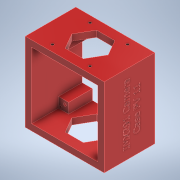
# Autodesk Inventor part: IMX291 Camera Case Base
Saved by Autodesk Inventor 2022.1 (Build 261234000, 234)
## iProperties
Created: 2021-07-23
Part Number: IMX291 Camera Case Base
Material: PET Plastic
Document SubType Name: Modeling
Designer: robst
Density: 1.541 g/cm^3
Appearance: Red
Author: robst
Autodesk Inventor part; units mm, degrees
ref_plane "YZ Plane" through (0, 0, 0) normal (1, 0, 0) x (0, 1, 0)
ref_plane "XZ Plane" through (0, 0, 0) normal (0, 1, 0) x (-1, 0, 0)
ref_plane "XY Plane" through (0, 0, 0) normal (0, 0, 1) x (1, 0, 0)
sketch "Sketch8" plane through (0, 0, 0) normal (0, 0, 1) x (1, 0, 0)
  line L0 (-17, -17) -> (17, -17) construction
  line L1 (17, -17) -> (17, 17) construction
  line L2 (17, 17) -> (-17, 17) construction
  line L3 (-17, 17) -> (-17, -17) construction
  line L4 (-17, -17) -> (17, 17) construction
  line L5 (17, -17) -> (-17, 17) construction
  circle A0 centre (-17, 17) radius 0.9
  circle A1 centre (17, 17) radius 0.9
  circle A2 centre (17, -17) radius 0.9
  circle A3 centre (-17, -17) radius 0.9
  line L6 (-21, -21) -> (21, -21)
  line L7 (21, -21) -> (21, 21)
  line L8 (21, 21) -> (-21, 21)
  line L9 (-21, 21) -> (-21, -21)
  line L10 (-21, -21) -> (21, 21) construction
  line L11 (21, -21) -> (-21, 21) construction
  line L12 (-25, -25) -> (25, -25)
  line L13 (25, -25) -> (25, 25)
  line L14 (25, 25) -> (-25, 25)
  line L15 (-25, 25) -> (-25, -25)
  line L16 (-25, -25) -> (25, 25) construction
  line L17 (25, -25) -> (-25, 25) construction
  line L18 (0, 0) -> (9.8286, 0)
  line L19 (-14.5, -14.5) -> (14.5, -14.5) construction
  line L20 (14.5, -14.5) -> (14.5, 14.5) construction
  line L21 (14.5, 14.5) -> (-14.5, 14.5) construction
  line L22 (-14.5, 14.5) -> (-14.5, -14.5) construction
  line L23 (-14.5, -14.5) -> (14.5, 14.5) construction
  line L24 (14.5, -14.5) -> (-14.5, 14.5) construction
  line L25 (-21, 21) -> (-14.5, 21)
  line L26 (-14.5, 21) -> (-14.5, 14.5)
  line L27 (-14.5, 14.5) -> (-21, 14.5)
  line L28 (-21, 14.5) -> (-21, 21)
  line L29 (21, 21) -> (14.5, 21)
  line L30 (14.5, 21) -> (14.5, 14.5)
  line L31 (14.5, 14.5) -> (21, 14.5)
  line L32 (21, 14.5) -> (21, 21)
  line L33 (21, -21) -> (14.5, -21)
  line L34 (14.5, -21) -> (14.5, -14.5)
  line L35 (14.5, -14.5) -> (21, -14.5)
  line L36 (21, -14.5) -> (21, -21)
  line L37 (-21, -21) -> (-14.5, -21)
  line L38 (-14.5, -21) -> (-14.5, -14.5)
  line L39 (-14.5, -14.5) -> (-21, -14.5)
  line L40 (-21, -14.5) -> (-21, -21)
  point P0 (-25, 0)
  point P1 (-14.5, -21)
  dimension "d46" = 34
  dimension "d47" = 34
  dimension "d48" = 1.8
  dimension "d49" = 42
  dimension "d50" = 42
  dimension "d51" = 4
  dimension "d52" = 4
  dimension "d53" = 29
  dimension "d54" = 29
  dimension "d61" = 50
  dimension "d62" = 50
  constraints: 82 end point, 16 parallel, 9 midpoint, 8 horizontal, 8 perpendicular, 4 centre point, 4 coincident, 3 equal radius, 2 point on line
  measures "d46" distance of L0.start L0.end
  measures "d47" distance of L2.end L0.start
  measures "d48" diameter of A0
  measures "d49" distance of L7.end L8.end
  measures "d50" distance of L6.end L7.end
  measures "d51" distance between parallel lines of L8 L14
  measures "d52" distance from line of point (-25, 0) L9
  measures "d53" distance of L19.start L19.end
  measures "d54" distance of L20.end L19.end
  measures "d61" distance between parallel lines of L14 L12
  measures "d62" distance between parallel lines of L15 L13
extrude "Extrusion9" add sketch "Sketch8" against normal blind 15 contours L9 L39 L38 L6 | L34 L35 L7 L6 | L9 L8 L26 L27 | L31 L30 L8 L7 | L15 L14 L13 L12
sketch "Sketch9" plane through (0, 0, 0) normal (0, 0, 1) x (1, 0, 0)
  line L0 (21, 14.5) -> (21, -14.5) projected
  line L1 (-14.5, 21) -> (14.5, 21) projected
  line L2 (-21, -14.5) -> (-21, 14.5) projected
  line L3 (14.5, -21) -> (-14.5, -21) projected
  line L4 (-25, -25) -> (25, -25) projected
  line L5 (25, -25) -> (25, 25) projected
  line L6 (25, 25) -> (-25, 25) projected
  line L7 (-25, 25) -> (-25, -25) projected
  line L8 (-21, -21) -> (21, -21)
  line L9 (21, -21) -> (21, 21)
  line L10 (21, 21) -> (-21, 21)
  line L11 (-21, 21) -> (-21, -21)
  line L12 (-21, -21) -> (21, 21) construction
  line L13 (21, -21) -> (-21, 21) construction
  line L14 (-23, -23) -> (23, -23)
  line L15 (23, -23) -> (23, 23)
  line L16 (23, 23) -> (-23, 23)
  line L17 (-23, 23) -> (-23, -23)
  line L18 (-23, -23) -> (23, 23) construction
  line L19 (23, -23) -> (-23, 23) construction
  point P0 (0, 0)
  point P1 (-14.5, -21)
  constraints: 24 end point, 4 midpoint, 4 parallel, 2 perpendicular
extrude "Extrusion10" add sketch "Sketch9" along normal blind 17 contours L7 L6 L5 L4 | L17 L16 L15 L14
sketch "Sketch10" plane through (25, -25, -15) normal (1, 0, 0) x (0, 0, -1)
  line L0 (-32, 0) -> (0, 0) construction
  line L1 (-16, 0) -> (-16, 50) construction
  line L2 (0, 50) -> (-32, 50) construction
  line L3 (-16, 7.4068) -> (-16, 5.8574)
  line L4 (-16, 5.8574) -> (-16.4084, 5.8574)
  line L5 (-16.4084, 5.8574) -> (-16.4084, 6.3663)
  line L6 (-16.4084, 6.3663) -> (-19.5916, 6.3663)
  line L7 (-19.5916, 6.3663) -> (-19.5916, 5.8574)
  line L8 (-19.5916, 5.8574) -> (-20, 5.8574)
  line L9 (-20, 5.8574) -> (-20, 7.4068)
  line L10 (-20, 7.4068) -> (-19.5916, 7.4068)
  line L11 (-19.5916, 7.4068) -> (-19.5916, 6.8979)
  line L12 (-19.5916, 6.8979) -> (-16.4084, 6.8979)
  line L13 (-16.4084, 6.8979) -> (-16.4084, 7.4068)
  line L14 (-16.4084, 7.4068) -> (-16, 7.4068)
  line L15 (-16, 11.4943) -> (-16, 10.9627)
  line L16 (-16, 10.9627) -> (-19.4457, 10.9627)
  line L17 (-19.4457, 10.9627) -> (-17.1021, 9.919)
  line L18 (-17.1021, 9.919) -> (-17.1021, 9.5948)
  line L19 (-17.1021, 9.5948) -> (-19.4457, 8.5608)
  line L20 (-19.4457, 8.5608) -> (-16, 8.5608)
  line L21 (-16, 8.5608) -> (-16, 8.0648)
  line L22 (-16, 8.0648) -> (-20, 8.0648)
  line L23 (-20, 8.0648) -> (-20, 8.7909)
  line L24 (-20, 8.7909) -> (-17.7731, 9.7893)
  line L25 (-17.7731, 9.7893) -> (-20, 10.7553)
  line L26 (-20, 10.7553) -> (-20, 11.4943)
  line L27 (-20, 11.4943) -> (-16, 11.4943)
  line L28 (-16, 15.0697) -> (-16, 14.4603)
  line L29 (-16, 14.4603) -> (-17.5948, 13.4878)
  line L30 (-17.5948, 13.4878) -> (-16, 12.4959)
  line L31 (-16, 12.4959) -> (-16, 11.9222)
  line L32 (-16, 11.9222) -> (-18.0032, 13.1961)
  line L33 (-18.0032, 13.1961) -> (-20, 11.9611)
  line L34 (-20, 11.9611) -> (-20, 12.5705)
  line L35 (-20, 12.5705) -> (-18.4344, 13.5235)
  line L36 (-18.4344, 13.5235) -> (-20, 14.4959)
  line L37 (-20, 14.4959) -> (-20, 15.0697)
  line L38 (-20, 15.0697) -> (-18.0292, 13.8185)
  line L39 (-18.0292, 13.8185) -> (-16, 15.0697)
  line L40 (-16, 17.8509) -> (-16, 15.3841)
  line L41 (-16, 15.3841) -> (-16.5673, 15.3841)
  spline S0 degree 2 poles (-16.5673, 15.3841) (-16.8169, 15.6499) (-17.2804, 16.1232) (-17.53, 16.3501) knots 0 0 0 1 2 2 2
  spline S1 degree 2 poles (-17.53, 16.3501) (-18.0324, 16.8071) (-18.6353, 17.141) (-18.9562, 17.141) knots 0 0 0 1 2 2 2
  spline S2 degree 2 poles (-18.9562, 17.141) (-19.1248, 17.141) (-19.3776, 17.0373) (-19.4587, 16.9433) knots 0 0 0 1 2 2 2
  spline S3 degree 2 poles (-19.4587, 16.9433) (-19.5397, 16.8493) (-19.6207, 16.6029) (-19.6207, 16.4538) knots 0 0 0 1 2 2 2
  spline S4 degree 2 poles (-19.6207, 16.4538) (-19.6207, 16.3112) (-19.5494, 16.0194) (-19.4943, 15.8865) knots 0 0 0 1 2 2 2
  spline S5 degree 2 poles (-19.4943, 15.8865) (-19.4489, 15.7731) (-19.3193, 15.5624) (-19.2739, 15.4976) knots 0 0 0 1 2 2 2
  line L42 (-19.2739, 15.4976) -> (-19.2739, 15.4684)
  line L43 (-19.2739, 15.4684) -> (-19.8444, 15.4684)
  spline S6 degree 2 poles (-19.8444, 15.4684) (-19.9254, 15.6337) (-20.0843, 16.2269) (-20.0843, 16.4927) knots 0 0 0 1 2 2 2
  spline S7 degree 2 poles (-20.0843, 16.4927) (-20.0843, 17.0535) (-19.4911, 17.6856) (-18.9854, 17.6856) knots 0 0 0 1 2 2 2
  spline S8 degree 2 poles (-18.9854, 17.6856) (-18.7488, 17.6856) (-18.3533, 17.5754) (-18.1848, 17.4781) knots 0 0 0 1 2 2 2
  spline S9 degree 2 poles (-18.1848, 17.4781) (-18.0097, 17.3809) (-17.6661, 17.0989) (-17.5008, 16.9433) knots 0 0 0 1 2 2 2
  spline S10 degree 2 poles (-17.5008, 16.9433) (-17.2253, 16.6904) (-16.6353, 16.0713) (-16.4635, 15.8865) knots 0 0 0 1 2 2 2
  line L44 (-16.4635, 15.8865) -> (-16.4635, 17.8509)
  line L45 (-16.4635, 17.8509) -> (-16, 17.8509)
  spline S11 degree 2 poles (-18.7002, 18.2755) (-19.0081, 18.2755) (-19.5203, 18.4765) (-19.705, 18.6515) knots 0 0 0 1 2 2 2
  spline S12 degree 2 poles (-19.705, 18.6515) (-19.8833, 18.8169) (-20.081, 19.2998) (-20.081, 19.5462) knots 0 0 0 1 2 2 2
  spline S13 degree 2 poles (-20.081, 19.5462) (-20.081, 19.8217) (-19.8963, 20.269) (-19.7212, 20.4344) knots 0 0 0 1 2 2 2
  spline S14 degree 2 poles (-19.7212, 20.4344) (-19.5008, 20.6418) (-18.7877, 20.8687) (-18.2399, 20.8687) knots 0 0 0 1 2 2 2
  spline S15 degree 2 poles (-18.2399, 20.8687) (-17.7439, 20.8687) (-16.8558, 20.6451) (-16.5608, 20.4279) knots 0 0 0 1 2 2 2
  spline S16 degree 2 poles (-16.5608, 20.4279) (-16.2496, 20.1977) (-15.9222, 19.5494) (-15.9222, 19.0762) knots 0 0 0 1 2 2 2
  spline S17 degree 2 poles (-15.9222, 19.0762) (-15.9222, 18.9692) (-15.9449, 18.7261) (-15.9773, 18.6224) knots 0 0 0 1 2 2 2
  line L46 (-15.9773, 18.6224) -> (-16.4927, 18.6224)
  line L47 (-16.4927, 18.6224) -> (-16.4927, 18.6483)
  spline S18 degree 2 poles (-16.4927, 18.6483) (-16.4538, 18.7164) (-16.3857, 19.0016) (-16.3857, 19.1475) knots 0 0 0 1 2 2 2
  spline S19 degree 2 poles (-16.3857, 19.1475) (-16.3857, 19.6726) (-17.0794, 20.2723) (-17.7212, 20.3144) knots 0 0 0 1 2 2 2
  spline S20 degree 2 poles (-17.7212, 20.3144) (-17.5754, 20.1005) (-17.4425, 19.7115) (-17.4425, 19.4814) knots 0 0 0 1 2 2 2
  spline S21 degree 2 poles (-17.4425, 19.4814) (-17.4425, 19.2609) (-17.5397, 18.8947) (-17.6791, 18.7099) knots 0 0 0 1 2 2 2
  spline S22 degree 2 poles (-17.6791, 18.7099) (-17.8444, 18.4959) (-18.3468, 18.2755) (-18.7002, 18.2755) knots 0 0 0 1 2 2 2
  spline S23 degree 2 poles (-18.3598, 20.3274) (-18.765, 20.3274) (-19.2771, 20.1783) (-19.4165, 20.0454) knots 0 0 0 1 2 2 2
  spline S24 degree 2 poles (-19.4165, 20.0454) (-19.5462, 19.9287) (-19.6434, 19.6856) (-19.6434, 19.5429) knots 0 0 0 1 2 2 2
  spline S25 degree 2 poles (-19.6434, 19.5429) (-19.6434, 19.2123) (-19.1702, 18.8201) (-18.7229, 18.8201) knots 0 0 0 1 2 2 2
  spline S26 degree 2 poles (-18.7229, 18.8201) (-18.47, 18.8201) (-18.1426, 18.9498) (-18.0259, 19.0924) knots 0 0 0 1 2 2 2
  spline S27 degree 2 poles (-18.0259, 19.0924) (-17.9417, 19.1961) (-17.8865, 19.4522) (-17.8865, 19.6013) knots 0 0 0 1 2 2 2
  spline S28 degree 2 poles (-17.8865, 19.6013) (-17.8865, 19.7731) (-18.0065, 20.1686) (-18.107, 20.3177) knots 0 0 0 1 2 2 2
  spline S29 degree 2 poles (-18.107, 20.3177) (-18.1459, 20.3209) (-18.2788, 20.3274) (-18.3598, 20.3274) knots 0 0 0 1 2 2 2
  line L48 (-16, 23.6532) -> (-16, 21.7018)
  line L49 (-16, 21.7018) -> (-16.4084, 21.7018)
  line L50 (-16.4084, 21.7018) -> (-16.4084, 22.4279)
  line L51 (-16.4084, 22.4279) -> (-19.0891, 22.4279)
  line L52 (-19.0891, 22.4279) -> (-19.0891, 21.7018)
  line L53 (-19.0891, 21.7018) -> (-19.4554, 21.7018)
  spline S30 degree 2 poles (-19.4554, 21.7018) (-19.4554, 22.1135) (-19.6888, 22.5024) (-20.013, 22.5284) knots 0 0 0 1 2 2 2
  line L54 (-20.013, 22.5284) -> (-20.013, 22.9433)
  line L55 (-20.013, 22.9433) -> (-16.4084, 22.9433)
  line L56 (-16.4084, 22.9433) -> (-16.4084, 23.6532)
  line L57 (-16.4084, 23.6532) -> (-16, 23.6532)
  spline S31 degree 2 poles (-15.9287, 27.7828) (-15.9287, 27.3938) (-16.1912, 26.7358) (-16.4538, 26.4959) knots 0 0 0 1 2 2 2
  spline S32 degree 2 poles (-16.4538, 26.4959) (-16.7131, 26.2561) (-17.4911, 25.9935) (-17.9968, 25.9935) knots 0 0 0 1 2 2 2
  spline S33 degree 2 poles (-17.9968, 25.9935) (-18.4992, 25.9935) (-19.2447, 26.2496) (-19.5203, 26.4927) knots 0 0 0 1 2 2 2
  spline S34 degree 2 poles (-19.5203, 26.4927) (-19.7893, 26.7326) (-20.0713, 27.3874) (-20.0713, 27.7925) knots 0 0 0 1 2 2 2
  spline S35 degree 2 poles (-20.0713, 27.7925) (-20.0713, 27.9935) (-20.013, 28.3468) (-19.9676, 28.4959) knots 0 0 0 1 2 2 2
  spline S36 degree 2 poles (-19.9676, 28.4959) (-19.9254, 28.6256) (-19.8055, 28.8947) (-19.7342, 29.0276) knots 0 0 0 1 2 2 2
  line L58 (-19.7342, 29.0276) -> (-19.0924, 29.0276)
  line L59 (-19.0924, 29.0276) -> (-19.0924, 28.9854)
  spline S37 degree 2 poles (-19.0924, 28.9854) (-19.1572, 28.9141) (-19.3387, 28.6937) (-19.4263, 28.5348) knots 0 0 0 1 2 2 2
  spline S38 degree 2 poles (-19.4263, 28.5348) (-19.5105, 28.3825) (-19.6175, 28.0227) (-19.6175, 27.7893) knots 0 0 0 1 2 2 2
  spline S39 degree 2 poles (-19.6175, 27.7893) (-19.6175, 27.5332) (-19.4068, 27.0762) (-19.2058, 26.9044) knots 0 0 0 1 2 2 2
  spline S40 degree 2 poles (-19.2058, 26.9044) (-19.0016, 26.7358) (-18.3825, 26.5478) (-17.9968, 26.5478) knots 0 0 0 1 2 2 2
  spline S41 degree 2 poles (-17.9968, 26.5478) (-17.5851, 26.5478) (-16.9919, 26.7455) (-16.7877, 26.9173) knots 0 0 0 1 2 2 2
  spline S42 degree 2 poles (-16.7877, 26.9173) (-16.59, 27.0859) (-16.389, 27.5365) (-16.389, 27.7893) knots 0 0 0 1 2 2 2
  spline S43 degree 2 poles (-16.389, 27.7893) (-16.389, 28.0194) (-16.5024, 28.4117) (-16.5867, 28.564) knots 0 0 0 1 2 2 2
  spline S44 degree 2 poles (-16.5867, 28.564) (-16.671, 28.7099) (-16.846, 28.9271) (-16.9076, 28.9887) knots 0 0 0 1 2 2 2
  line L60 (-16.9076, 28.9887) -> (-16.9076, 29.0276)
  line L61 (-16.9076, 29.0276) -> (-16.2723, 29.0276)
  spline S45 degree 2 poles (-16.2723, 29.0276) (-16.2107, 28.8947) (-16.0972, 28.6613) (-16.0454, 28.4959) knots 0 0 0 1 2 2 2
  spline S46 degree 2 poles (-16.0454, 28.4959) (-15.987, 28.3209) (-15.9287, 28.0227) (-15.9287, 27.7828) knots 0 0 0 1 2 2 2
  spline S47 degree 2 poles (-16.3177, 31.1572) (-16.2723, 31.0956) (-16.1102, 30.8882) (-16.0616, 30.7909) knots 0 0 0 1 2 2 2
  spline S48 degree 2 poles (-16.0616, 30.7909) (-15.9903, 30.658) (-15.9157, 30.4084) (-15.9157, 30.1815) knots 0 0 0 1 2 2 2
  spline S49 degree 2 poles (-15.9157, 30.1815) (-15.9157, 29.9968) (-16.0551, 29.6629) (-16.1815, 29.5365) knots 0 0 0 1 2 2 2
  spline S50 degree 2 poles (-16.1815, 29.5365) (-16.3047, 29.4165) (-16.6677, 29.2707) (-16.8687, 29.2707) knots 0 0 0 1 2 2 2
  spline S51 degree 2 poles (-16.8687, 29.2707) (-17.1799, 29.2707) (-17.6207, 29.5332) (-17.7472, 29.8185) knots 0 0 0 1 2 2 2
  spline S52 degree 2 poles (-17.7472, 29.8185) (-17.8639, 30.0713) (-17.9514, 30.7585) (-17.9741, 31.1572) knots 0 0 0 1 2 2 2
  line L62 (-17.9741, 31.1572) -> (-18.0713, 31.1572)
  spline S53 degree 2 poles (-18.0713, 31.1572) (-18.2464, 31.1572) (-18.4635, 31.0502) (-18.5251, 30.953) knots 0 0 0 1 2 2 2
  spline S54 degree 2 poles (-18.5251, 30.953) (-18.5867, 30.8558) (-18.6256, 30.577) (-18.6256, 30.4279) knots 0 0 0 1 2 2 2
  spline S55 degree 2 poles (-18.6256, 30.4279) (-18.6256, 30.2528) (-18.5219, 29.7796) (-18.4214, 29.543) knots 0 0 0 1 2 2 2
  line L63 (-18.4214, 29.543) -> (-18.4214, 29.5138)
  line L64 (-18.4214, 29.5138) -> (-18.9368, 29.5138)
  spline S56 degree 2 poles (-18.9368, 29.5138) (-18.9757, 29.6532) (-19.0729, 30.175) (-19.0729, 30.4311) knots 0 0 0 1 2 2 2
  spline S57 degree 2 poles (-19.0729, 30.4311) (-19.0729, 30.7423) (-18.9757, 31.1669) (-18.8493, 31.3355) knots 0 0 0 1 2 2 2
  spline S58 degree 2 poles (-18.8493, 31.3355) (-18.7261, 31.5008) (-18.3339, 31.6629) (-18.0519, 31.6629) knots 0 0 0 1 2 2 2
  line L65 (-18.0519, 31.6629) -> (-16, 31.6629)
  line L66 (-16, 31.6629) -> (-16, 31.1572)
  line L67 (-16, 31.1572) -> (-16.3177, 31.1572)
  line L68 (-16.7391, 31.1572) -> (-17.5721, 31.1572)
  spline S59 degree 2 poles (-17.5721, 31.1572) (-17.5559, 30.9757) (-17.5008, 30.4279) (-17.4489, 30.2561) knots 0 0 0 1 2 2 2
  spline S60 degree 2 poles (-17.4489, 30.2561) (-17.3874, 30.0551) (-17.1313, 29.7925) (-16.9044, 29.7925) knots 0 0 0 1 2 2 2
  spline S61 degree 2 poles (-16.9044, 29.7925) (-16.6451, 29.7925) (-16.3825, 30.0843) (-16.3825, 30.363) knots 0 0 0 1 2 2 2
  spline S62 degree 2 poles (-16.3825, 30.363) (-16.3825, 30.5997) (-16.5867, 30.9887) (-16.7391, 31.1572) knots 0 0 0 1 2 2 2
  line L69 (-16, 35.7763) -> (-17.7374, 35.7763)
  spline S63 degree 2 poles (-17.7374, 35.7763) (-17.9449, 35.7763) (-18.2982, 35.7439) (-18.3955, 35.6921) knots 0 0 0 1 2 2 2
  spline S64 degree 2 poles (-18.3955, 35.6921) (-18.5024, 35.6402) (-18.6062, 35.4425) (-18.6062, 35.2707) knots 0 0 0 1 2 2 2
  spline S65 degree 2 poles (-18.6062, 35.2707) (-18.6062, 35.1151) (-18.4149, 34.7585) (-18.2334, 34.5705) knots 0 0 0 1 2 2 2
  spline S66 degree 2 poles (-18.2334, 34.5705) (-18.188, 34.5737) (-18.0616, 34.5802) (-17.9773, 34.5802) knots 0 0 0 1 2 2 2
  line L70 (-17.9773, 34.5802) -> (-16, 34.5802)
  line L71 (-16, 34.5802) -> (-16, 34.0746)
  line L72 (-16, 34.0746) -> (-17.7374, 34.0746)
  spline S67 degree 2 poles (-17.7374, 34.0746) (-17.9449, 34.0746) (-18.2982, 34.0421) (-18.3955, 33.9903) knots 0 0 0 1 2 2 2
  spline S68 degree 2 poles (-18.3955, 33.9903) (-18.5024, 33.9384) (-18.6062, 33.7407) (-18.6062, 33.5689) knots 0 0 0 1 2 2 2
  spline S69 degree 2 poles (-18.6062, 33.5689) (-18.6062, 33.4068) (-18.4019, 33.047) (-18.2431, 32.8784) knots 0 0 0 1 2 2 2
  line L73 (-18.2431, 32.8784) -> (-16, 32.8784)
  line L74 (-16, 32.8784) -> (-16, 32.3728)
  line L75 (-16, 32.3728) -> (-19.0016, 32.3728)
  line L76 (-19.0016, 32.3728) -> (-19.0016, 32.8784)
  line L77 (-19.0016, 32.8784) -> (-18.671, 32.8784)
  spline S70 degree 2 poles (-18.671, 32.8784) (-18.8687, 33.0762) (-19.0859, 33.4652) (-19.0859, 33.6985) knots 0 0 0 1 2 2 2
  spline S71 degree 2 poles (-19.0859, 33.6985) (-19.0859, 33.9643) (-18.8428, 34.376) (-18.5673, 34.483) knots 0 0 0 1 2 2 2
  spline S72 degree 2 poles (-18.5673, 34.483) (-18.8233, 34.7131) (-19.0859, 35.1475) (-19.0859, 35.4003) knots 0 0 0 1 2 2 2
  spline S73 degree 2 poles (-19.0859, 35.4003) (-19.0859, 35.5948) (-18.966, 35.9125) (-18.8298, 36.0292) knots 0 0 0 1 2 2 2
  spline S74 degree 2 poles (-18.8298, 36.0292) (-18.6937, 36.1491) (-18.2853, 36.282) (-17.9773, 36.282) knots 0 0 0 1 2 2 2
  line L78 (-17.9773, 36.282) -> (-16, 36.282)
  line L79 (-16, 36.282) -> (-16, 35.7763)
  spline S75 degree 2 poles (-15.9319, 38.295) (-15.9319, 37.5754) (-16.7391, 36.7844) (-17.4846, 36.7844) knots 0 0 0 1 2 2 2
  spline S76 degree 2 poles (-17.4846, 36.7844) (-18.2172, 36.7844) (-19.0859, 37.5527) (-19.0859, 38.1718) knots 0 0 0 1 2 2 2
  spline S77 degree 2 poles (-19.0859, 38.1718) (-19.0859, 38.4506) (-18.9238, 38.8817) (-18.752, 39.0405) knots 0 0 0 1 2 2 2
  spline S78 degree 2 poles (-18.752, 39.0405) (-18.5802, 39.2026) (-18.0843, 39.3744) (-17.7245, 39.3744) knots 0 0 0 1 2 2 2
  line L80 (-17.7245, 39.3744) -> (-17.4489, 39.3744)
  line L81 (-17.4489, 39.3744) -> (-17.4489, 37.2966)
  spline S79 degree 2 poles (-17.4489, 37.2966) (-16.9271, 37.2966) (-16.3728, 37.8217) (-16.3728, 38.2885) knots 0 0 0 1 2 2 2
  spline S80 degree 2 poles (-16.3728, 38.2885) (-16.3728, 38.4538) (-16.4473, 38.7747) (-16.5057, 38.9044) knots 0 0 0 1 2 2 2
  spline S81 degree 2 poles (-16.5057, 38.9044) (-16.5705, 39.0405) (-16.684, 39.2285) (-16.7358, 39.2901) knots 0 0 0 1 2 2 2
  line L82 (-16.7358, 39.2901) -> (-16.7358, 39.3193)
  line L83 (-16.7358, 39.3193) -> (-16.1848, 39.3193)
  spline S82 degree 2 poles (-16.1848, 39.3193) (-16.1491, 39.2318) (-16.0454, 38.966) (-16.0162, 38.8622) knots 0 0 0 1 2 2 2
  spline S83 degree 2 poles (-16.0162, 38.8622) (-15.9741, 38.7164) (-15.9319, 38.4765) (-15.9319, 38.295) knots 0 0 0 1 2 2 2
  spline S84 degree 2 poles (-17.8347, 38.8817) (-18.0389, 38.8752) (-18.3371, 38.7909) (-18.4376, 38.7099) knots 0 0 0 1 2 2 2
  spline S85 degree 2 poles (-18.4376, 38.7099) (-18.5511, 38.6224) (-18.671, 38.3468) (-18.671, 38.1426) knots 0 0 0 1 2 2 2
  spline S86 degree 2 poles (-18.671, 38.1426) (-18.671, 37.9417) (-18.5511, 37.6596) (-18.4344, 37.543) knots 0 0 0 1 2 2 2
  spline S87 degree 2 poles (-18.4344, 37.543) (-18.3144, 37.4295) (-18.0259, 37.3128) (-17.8347, 37.2966) knots 0 0 0 1 2 2 2
  line L84 (-17.8347, 37.2966) -> (-17.8347, 38.8817)
  line L85 (-18.4603, 41.4781) -> (-18.4603, 41.4522)
  spline S88 degree 2 poles (-18.4603, 41.4522) (-18.4765, 41.3938) (-18.483, 41.2674) (-18.483, 41.1799) knots 0 0 0 1 2 2 2
  spline S89 degree 2 poles (-18.483, 41.1799) (-18.483, 40.9757) (-18.3047, 40.5737) (-18.1297, 40.3922) knots 0 0 0 1 2 2 2
  line L86 (-18.1297, 40.3922) -> (-16, 40.3922)
  line L87 (-16, 40.3922) -> (-16, 39.8865)
  line L88 (-16, 39.8865) -> (-19.0016, 39.8865)
  line L89 (-19.0016, 39.8865) -> (-19.0016, 40.3922)
  line L90 (-19.0016, 40.3922) -> (-18.5543, 40.3922)
  spline S90 degree 2 poles (-18.5543, 40.3922) (-18.8006, 40.6677) (-19.0016, 41.0794) (-19.0016, 41.2739) knots 0 0 0 1 2 2 2
  spline S91 degree 2 poles (-19.0016, 41.2739) (-19.0016, 41.3517) (-18.9951, 41.4295) (-18.9854, 41.4781) knots 0 0 0 1 2 2 2
  line L91 (-18.9854, 41.4781) -> (-18.4603, 41.4781)
  spline S92 degree 2 poles (-16.3177, 43.543) (-16.2723, 43.4814) (-16.1102, 43.2739) (-16.0616, 43.1767) knots 0 0 0 1 2 2 2
  spline S93 degree 2 poles (-16.0616, 43.1767) (-15.9903, 43.0438) (-15.9157, 42.7942) (-15.9157, 42.5673) knots 0 0 0 1 2 2 2
  spline S94 degree 2 poles (-15.9157, 42.5673) (-15.9157, 42.3825) (-16.0551, 42.0486) (-16.1815, 41.9222) knots 0 0 0 1 2 2 2
  spline S95 degree 2 poles (-16.1815, 41.9222) (-16.3047, 41.8023) (-16.6677, 41.6564) (-16.8687, 41.6564) knots 0 0 0 1 2 2 2
  spline S96 degree 2 poles (-16.8687, 41.6564) (-17.1799, 41.6564) (-17.6207, 41.919) (-17.7472, 42.2042) knots 0 0 0 1 2 2 2
  spline S97 degree 2 poles (-17.7472, 42.2042) (-17.8639, 42.4571) (-17.9514, 43.1442) (-17.9741, 43.543) knots 0 0 0 1 2 2 2
  line L92 (-17.9741, 43.543) -> (-18.0713, 43.543)
  spline S98 degree 2 poles (-18.0713, 43.543) (-18.2464, 43.543) (-18.4635, 43.436) (-18.5251, 43.3387) knots 0 0 0 1 2 2 2
  spline S99 degree 2 poles (-18.5251, 43.3387) (-18.5867, 43.2415) (-18.6256, 42.9627) (-18.6256, 42.8136) knots 0 0 0 1 2 2 2
  spline S100 degree 2 poles (-18.6256, 42.8136) (-18.6256, 42.6386) (-18.5219, 42.1653) (-18.4214, 41.9287) knots 0 0 0 1 2 2 2
  line L93 (-18.4214, 41.9287) -> (-18.4214, 41.8995)
  line L94 (-18.4214, 41.8995) -> (-18.9368, 41.8995)
  spline S101 degree 2 poles (-18.9368, 41.8995) (-18.9757, 42.0389) (-19.0729, 42.5608) (-19.0729, 42.8169) knots 0 0 0 1 2 2 2
  spline S102 degree 2 poles (-19.0729, 42.8169) (-19.0729, 43.128) (-18.9757, 43.5527) (-18.8493, 43.7212) knots 0 0 0 1 2 2 2
  spline S103 degree 2 poles (-18.8493, 43.7212) (-18.7261, 43.8865) (-18.3339, 44.0486) (-18.0519, 44.0486) knots 0 0 0 1 2 2 2
  line L95 (-18.0519, 44.0486) -> (-16, 44.0486)
  line L96 (-16, 44.0486) -> (-16, 43.543)
  line L97 (-16, 43.543) -> (-16.3177, 43.543)
  line L98 (-16.7391, 43.543) -> (-17.5721, 43.543)
  spline S104 degree 2 poles (-17.5721, 43.543) (-17.5559, 43.3614) (-17.5008, 42.8136) (-17.4489, 42.6418) knots 0 0 0 1 2 2 2
  spline S105 degree 2 poles (-17.4489, 42.6418) (-17.3874, 42.4408) (-17.1313, 42.1783) (-16.9044, 42.1783) knots 0 0 0 1 2 2 2
  spline S106 degree 2 poles (-16.9044, 42.1783) (-16.6451, 42.1783) (-16.3825, 42.47) (-16.3825, 42.7488) knots 0 0 0 1 2 2 2
  spline S107 degree 2 poles (-16.3825, 42.7488) (-16.3825, 42.9854) (-16.5867, 43.3744) (-16.7391, 43.543) knots 0 0 0 1 2 2 2
  spline S108 degree 2 poles (-9.3362, 13.3193) (-9.3362, 12.9303) (-9.5988, 12.2723) (-9.8613, 12.0324) knots 0 0 0 1 2 2 2
  spline S109 degree 2 poles (-9.8613, 12.0324) (-10.1207, 11.7925) (-10.8986, 11.53) (-11.4043, 11.53) knots 0 0 0 1 2 2 2
  spline S110 degree 2 poles (-11.4043, 11.53) (-11.9067, 11.53) (-12.6523, 11.7861) (-12.9278, 12.0292) knots 0 0 0 1 2 2 2
  spline S111 degree 2 poles (-12.9278, 12.0292) (-13.1968, 12.269) (-13.4788, 12.9238) (-13.4788, 13.329) knots 0 0 0 1 2 2 2
  spline S112 degree 2 poles (-13.4788, 13.329) (-13.4788, 13.53) (-13.4205, 13.8833) (-13.3751, 14.0324) knots 0 0 0 1 2 2 2
  spline S113 degree 2 poles (-13.3751, 14.0324) (-13.333, 14.1621) (-13.213, 14.4311) (-13.1417, 14.564) knots 0 0 0 1 2 2 2
  line L99 (-13.1417, 14.564) -> (-12.4999, 14.564)
  line L100 (-12.4999, 14.564) -> (-12.4999, 14.5219)
  spline S114 degree 2 poles (-12.4999, 14.5219) (-12.5647, 14.4506) (-12.7463, 14.2301) (-12.8338, 14.0713) knots 0 0 0 1 2 2 2
  spline S115 degree 2 poles (-12.8338, 14.0713) (-12.9181, 13.919) (-13.025, 13.5592) (-13.025, 13.3258) knots 0 0 0 1 2 2 2
  spline S116 degree 2 poles (-13.025, 13.3258) (-13.025, 13.0697) (-12.8143, 12.6126) (-12.6134, 12.4408) knots 0 0 0 1 2 2 2
  spline S117 degree 2 poles (-12.6134, 12.4408) (-12.4091, 12.2723) (-11.79, 12.0843) (-11.4043, 12.0843) knots 0 0 0 1 2 2 2
  spline S118 degree 2 poles (-11.4043, 12.0843) (-10.9926, 12.0843) (-10.3994, 12.282) (-10.1952, 12.4538) knots 0 0 0 1 2 2 2
  spline S119 degree 2 poles (-10.1952, 12.4538) (-9.9975, 12.6224) (-9.7965, 13.0729) (-9.7965, 13.3258) knots 0 0 0 1 2 2 2
  spline S120 degree 2 poles (-9.7965, 13.3258) (-9.7965, 13.5559) (-9.91, 13.9481) (-9.9942, 14.1005) knots 0 0 0 1 2 2 2
  spline S121 degree 2 poles (-9.9942, 14.1005) (-10.0785, 14.2464) (-10.2536, 14.4635) (-10.3151, 14.5251) knots 0 0 0 1 2 2 2
  line L101 (-10.3151, 14.5251) -> (-10.3151, 14.564)
  line L102 (-10.3151, 14.564) -> (-9.6798, 14.564)
  spline S122 degree 2 poles (-9.6798, 14.564) (-9.6182, 14.4311) (-9.5048, 14.1977) (-9.4529, 14.0324) knots 0 0 0 1 2 2 2
  spline S123 degree 2 poles (-9.4529, 14.0324) (-9.3946, 13.8574) (-9.3362, 13.5592) (-9.3362, 13.3193) knots 0 0 0 1 2 2 2
  spline S124 degree 2 poles (-9.7252, 16.6937) (-9.6798, 16.6321) (-9.5177, 16.4246) (-9.4691, 16.3274) knots 0 0 0 1 2 2 2
  spline S125 degree 2 poles (-9.4691, 16.3274) (-9.3978, 16.1945) (-9.3233, 15.9449) (-9.3233, 15.718) knots 0 0 0 1 2 2 2
  spline S126 degree 2 poles (-9.3233, 15.718) (-9.3233, 15.5332) (-9.4626, 15.1994) (-9.5891, 15.0729) knots 0 0 0 1 2 2 2
  spline S127 degree 2 poles (-9.5891, 15.0729) (-9.7122, 14.953) (-10.0753, 14.8071) (-10.2762, 14.8071) knots 0 0 0 1 2 2 2
  spline S128 degree 2 poles (-10.2762, 14.8071) (-10.5874, 14.8071) (-11.0283, 15.0697) (-11.1547, 15.3549) knots 0 0 0 1 2 2 2
  spline S129 degree 2 poles (-11.1547, 15.3549) (-11.2714, 15.6078) (-11.3589, 16.295) (-11.3816, 16.6937) knots 0 0 0 1 2 2 2
  line L103 (-11.3816, 16.6937) -> (-11.4788, 16.6937)
  spline S130 degree 2 poles (-11.4788, 16.6937) (-11.6539, 16.6937) (-11.8711, 16.5867) (-11.9327, 16.4895) knots 0 0 0 1 2 2 2
  spline S131 degree 2 poles (-11.9327, 16.4895) (-11.9942, 16.3922) (-12.0331, 16.1135) (-12.0331, 15.9643) knots 0 0 0 1 2 2 2
  spline S132 degree 2 poles (-12.0331, 15.9643) (-12.0331, 15.7893) (-11.9294, 15.316) (-11.8289, 15.0794) knots 0 0 0 1 2 2 2
  line L104 (-11.8289, 15.0794) -> (-11.8289, 15.0502)
  line L105 (-11.8289, 15.0502) -> (-12.3443, 15.0502)
  spline S133 degree 2 poles (-12.3443, 15.0502) (-12.3832, 15.1896) (-12.4805, 15.7115) (-12.4805, 15.9676) knots 0 0 0 1 2 2 2
  spline S134 degree 2 poles (-12.4805, 15.9676) (-12.4805, 16.2788) (-12.3832, 16.7034) (-12.2568, 16.872) knots 0 0 0 1 2 2 2
  spline S135 degree 2 poles (-12.2568, 16.872) (-12.1336, 17.0373) (-11.7414, 17.1994) (-11.4594, 17.1994) knots 0 0 0 1 2 2 2
  line L106 (-11.4594, 17.1994) -> (-9.4075, 17.1994)
  line L107 (-9.4075, 17.1994) -> (-9.4075, 16.6937)
  line L108 (-9.4075, 16.6937) -> (-9.7252, 16.6937)
  line L109 (-10.1466, 16.6937) -> (-10.9797, 16.6937)
  spline S136 degree 2 poles (-10.9797, 16.6937) (-10.9634, 16.5122) (-10.9083, 15.9643) (-10.8565, 15.7925) knots 0 0 0 1 2 2 2
  spline S137 degree 2 poles (-10.8565, 15.7925) (-10.7949, 15.5916) (-10.5388, 15.329) (-10.3119, 15.329) knots 0 0 0 1 2 2 2
  spline S138 degree 2 poles (-10.3119, 15.329) (-10.0526, 15.329) (-9.79, 15.6207) (-9.79, 15.8995) knots 0 0 0 1 2 2 2
  spline S139 degree 2 poles (-9.79, 15.8995) (-9.79, 16.1361) (-9.9942, 16.5251) (-10.1466, 16.6937) knots 0 0 0 1 2 2 2
  spline S140 degree 2 poles (-9.3362, 18.7196) (-9.3362, 18.4182) (-9.4983, 17.8963) (-9.5891, 17.7245) knots 0 0 0 1 2 2 2
  line L110 (-9.5891, 17.7245) -> (-10.1563, 17.7245)
  line L111 (-10.1563, 17.7245) -> (-10.1563, 17.7504)
  spline S141 degree 2 poles (-10.1563, 17.7504) (-10.1044, 17.8152) (-9.9813, 17.9903) (-9.9132, 18.1361) knots 0 0 0 1 2 2 2
  spline S142 degree 2 poles (-9.9132, 18.1361) (-9.8516, 18.2626) (-9.7609, 18.5737) (-9.7609, 18.7391) knots 0 0 0 1 2 2 2
  spline S143 degree 2 poles (-9.7609, 18.7391) (-9.7609, 18.859) (-9.816, 19.1345) (-9.8613, 19.1994) knots 0 0 0 1 2 2 2
  spline S144 degree 2 poles (-9.8613, 19.1994) (-9.9229, 19.2934) (-10.0623, 19.3776) (-10.2049, 19.3776) knots 0 0 0 1 2 2 2
  spline S145 degree 2 poles (-10.2049, 19.3776) (-10.3832, 19.3776) (-10.568, 19.1831) (-10.6296, 18.9335) knots 0 0 0 1 2 2 2
  spline S146 degree 2 poles (-10.6296, 18.9335) (-10.6523, 18.8363) (-10.7171, 18.5251) (-10.7527, 18.3922) knots 0 0 0 1 2 2 2
  spline S147 degree 2 poles (-10.7527, 18.3922) (-10.8532, 18.0486) (-11.2681, 17.7374) (-11.5631, 17.7374) knots 0 0 0 1 2 2 2
  spline S148 degree 2 poles (-11.5631, 17.7374) (-11.9715, 17.7374) (-12.4805, 18.3501) (-12.4805, 18.8558) knots 0 0 0 1 2 2 2
  spline S149 degree 2 poles (-12.4805, 18.8558) (-12.4805, 19.1053) (-12.3573, 19.611) (-12.2633, 19.7828) knots 0 0 0 1 2 2 2
  line L112 (-12.2633, 19.7828) -> (-11.722, 19.7828)
  line L113 (-11.722, 19.7828) -> (-11.722, 19.7569)
  spline S150 degree 2 poles (-11.722, 19.7569) (-11.8775, 19.5624) (-12.0558, 19.0891) (-12.0558, 18.846) knots 0 0 0 1 2 2 2
  spline S151 degree 2 poles (-12.0558, 18.846) (-12.0558, 18.5964) (-11.8451, 18.2528) (-11.6344, 18.2528) knots 0 0 0 1 2 2 2
  spline S152 degree 2 poles (-11.6344, 18.2528) (-11.4432, 18.2528) (-11.2584, 18.457) (-11.2001, 18.684) knots 0 0 0 1 2 2 2
  spline S153 degree 2 poles (-11.2001, 18.684) (-11.1709, 18.7942) (-11.1126, 19.0729) (-11.0769, 19.2253) knots 0 0 0 1 2 2 2
  spline S154 degree 2 poles (-11.0769, 19.2253) (-10.9926, 19.5559) (-10.6069, 19.893) (-10.273, 19.893) knots 0 0 0 1 2 2 2
  spline S155 degree 2 poles (-10.273, 19.893) (-10.0785, 19.893) (-9.7349, 19.7407) (-9.6085, 19.5916) knots 0 0 0 1 2 2 2
  spline S156 degree 2 poles (-9.6085, 19.5916) (-9.4756, 19.4327) (-9.3362, 19.0276) (-9.3362, 18.7196) knots 0 0 0 1 2 2 2
  spline S157 degree 2 poles (-9.3395, 21.6661) (-9.3395, 20.9465) (-10.1466, 20.1556) (-10.8921, 20.1556) knots 0 0 0 1 2 2 2
  spline S158 degree 2 poles (-10.8921, 20.1556) (-11.6247, 20.1556) (-12.4934, 20.9238) (-12.4934, 21.5429) knots 0 0 0 1 2 2 2
  spline S159 degree 2 poles (-12.4934, 21.5429) (-12.4934, 21.8217) (-12.3314, 22.2528) (-12.1596, 22.4117) knots 0 0 0 1 2 2 2
  spline S160 degree 2 poles (-12.1596, 22.4117) (-11.9878, 22.5737) (-11.4918, 22.7455) (-11.132, 22.7455) knots 0 0 0 1 2 2 2
  line L114 (-11.132, 22.7455) -> (-10.8565, 22.7455)
  line L115 (-10.8565, 22.7455) -> (-10.8565, 20.6677)
  spline S161 degree 2 poles (-10.8565, 20.6677) (-10.3346, 20.6677) (-9.7803, 21.1929) (-9.7803, 21.6596) knots 0 0 0 1 2 2 2
  spline S162 degree 2 poles (-9.7803, 21.6596) (-9.7803, 21.825) (-9.8549, 22.1459) (-9.9132, 22.2755) knots 0 0 0 1 2 2 2
  spline S163 degree 2 poles (-9.9132, 22.2755) (-9.978, 22.4117) (-10.0915, 22.5997) (-10.1433, 22.6613) knots 0 0 0 1 2 2 2
  line L116 (-10.1433, 22.6613) -> (-10.1433, 22.6904)
  line L117 (-10.1433, 22.6904) -> (-9.5923, 22.6904)
  spline S164 degree 2 poles (-9.5923, 22.6904) (-9.5566, 22.6029) (-9.4529, 22.3371) (-9.4237, 22.2334) knots 0 0 0 1 2 2 2
  spline S165 degree 2 poles (-9.4237, 22.2334) (-9.3816, 22.0875) (-9.3395, 21.8476) (-9.3395, 21.6661) knots 0 0 0 1 2 2 2
  spline S166 degree 2 poles (-11.2422, 22.2528) (-11.4464, 22.2464) (-11.7446, 22.1621) (-11.8451, 22.081) knots 0 0 0 1 2 2 2
  spline S167 degree 2 poles (-11.8451, 22.081) (-11.9586, 21.9935) (-12.0785, 21.718) (-12.0785, 21.5138) knots 0 0 0 1 2 2 2
  spline S168 degree 2 poles (-12.0785, 21.5138) (-12.0785, 21.3128) (-11.9586, 21.0308) (-11.8419, 20.9141) knots 0 0 0 1 2 2 2
  spline S169 degree 2 poles (-11.8419, 20.9141) (-11.722, 20.8006) (-11.4335, 20.684) (-11.2422, 20.6677) knots 0 0 0 1 2 2 2
  line L118 (-11.2422, 20.6677) -> (-11.2422, 22.2528)
  spline S170 degree 2 poles (-12.2017, 27.5429) (-11.9424, 27.5429) (-11.4756, 27.3582) (-11.3135, 27.1929) knots 0 0 0 1 2 2 2
  spline S171 degree 2 poles (-11.3135, 27.1929) (-11.1093, 26.9854) (-10.8986, 26.4246) (-10.8986, 25.9968) knots 0 0 0 1 2 2 2
  line L119 (-10.8986, 25.9968) -> (-10.8986, 25.5462)
  line L120 (-10.8986, 25.5462) -> (-9.4075, 25.5462)
  line L121 (-9.4075, 25.5462) -> (-9.4075, 25.0146)
  line L122 (-9.4075, 25.0146) -> (-13.4075, 25.0146)
  line L123 (-13.4075, 25.0146) -> (-13.4075, 26.0194)
  spline S172 degree 2 poles (-13.4075, 26.0194) (-13.4075, 26.376) (-13.2908, 26.8752) (-13.1579, 27.0665) knots 0 0 0 1 2 2 2
  spline S173 degree 2 poles (-13.1579, 27.0665) (-13.0056, 27.2901) (-12.5356, 27.5429) (-12.2017, 27.5429) knots 0 0 0 1 2 2 2
  spline S174 degree 2 poles (-12.1855, 26.9887) (-12.3929, 26.9887) (-12.6976, 26.846) (-12.7949, 26.7002) knots 0 0 0 1 2 2 2
  spline S175 degree 2 poles (-12.7949, 26.7002) (-12.8792, 26.5737) (-12.9472, 26.2366) (-12.9472, 25.987) knots 0 0 0 1 2 2 2
  line L124 (-12.9472, 25.987) -> (-12.9472, 25.5462)
  line L125 (-12.9472, 25.5462) -> (-11.3524, 25.5462)
  line L126 (-11.3524, 25.5462) -> (-11.3524, 25.9092)
  spline S176 degree 2 poles (-11.3524, 25.9092) (-11.3524, 26.2334) (-11.4562, 26.6321) (-11.5923, 26.7618) knots 0 0 0 1 2 2 2
  spline S177 degree 2 poles (-11.5923, 26.7618) (-11.7122, 26.8817) (-11.9942, 26.9887) (-12.1855, 26.9887) knots 0 0 0 1 2 2 2
  line L127 (-13.4075, 30.9498) -> (-9.4075, 29.5721)
  line L128 (-9.4075, 29.5721) -> (-9.4075, 28.9984)
  line L129 (-9.4075, 28.9984) -> (-13.4075, 27.6207)
  line L130 (-13.4075, 27.6207) -> (-13.4075, 28.1912)
  line L131 (-13.4075, 28.1912) -> (-10.085, 29.2998)
  line L132 (-10.085, 29.2998) -> (-13.4075, 30.4084)
  line L133 (-13.4075, 30.4084) -> (-13.4075, 30.9498)
  line L134 (-9.4075, 35.248) -> (-9.4075, 33.2966)
  line L135 (-9.4075, 33.2966) -> (-9.816, 33.2966)
  line L136 (-9.816, 33.2966) -> (-9.816, 34.0227)
  line L137 (-9.816, 34.0227) -> (-12.4967, 34.0227)
  line L138 (-12.4967, 34.0227) -> (-12.4967, 33.2966)
  line L139 (-12.4967, 33.2966) -> (-12.863, 33.2966)
  spline S178 degree 2 poles (-12.863, 33.2966) (-12.863, 33.7083) (-13.0963, 34.0972) (-13.4205, 34.1232) knots 0 0 0 1 2 2 2
  line L140 (-13.4205, 34.1232) -> (-13.4205, 34.5381)
  line L141 (-13.4205, 34.5381) -> (-9.816, 34.5381)
  line L142 (-9.816, 34.5381) -> (-9.816, 35.248)
  line L143 (-9.816, 35.248) -> (-9.4075, 35.248)
  line L144 (-9.4075, 38.2496) -> (-9.4075, 36.2982)
  line L145 (-9.4075, 36.2982) -> (-9.816, 36.2982)
  line L146 (-9.816, 36.2982) -> (-9.816, 37.0243)
  line L147 (-9.816, 37.0243) -> (-12.4967, 37.0243)
  line L148 (-12.4967, 37.0243) -> (-12.4967, 36.2982)
  line L149 (-12.4967, 36.2982) -> (-12.863, 36.2982)
  spline S179 degree 2 poles (-12.863, 36.2982) (-12.863, 36.7099) (-13.0963, 37.0989) (-13.4205, 37.1248) knots 0 0 0 1 2 2 2
  line L150 (-13.4205, 37.1248) -> (-13.4205, 37.5397)
  line L151 (-13.4205, 37.5397) -> (-9.816, 37.5397)
  line L152 (-9.816, 37.5397) -> (-9.816, 38.2496)
  line L153 (-9.816, 38.2496) -> (-9.4075, 38.2496)
  point P0 (-15, 25)
  constraints: 2 end point, 2 midpoint, 1 vertical
emboss "Emboss2" sketch "Sketch10" operation cut depth 1 direction (-1, 0, 0)
sketch "Sketch11" plane through (0, 0, -15) normal (0, 0, -1) x (-1, 0, 0)
  line L0 (25, -25) -> (25, 25) projected
  line L1 (-25, -25) -> (25, -25) projected
  line L2 (-25, 25) -> (-25, -25) projected
  line L3 (25, 25) -> (-25, 25) projected
  line L4 (-19.75, 19.75) -> (-19.75, -19.75) construction
  line L5 (-19.75, -19.75) -> (19.75, -19.75) construction
  line L6 (19.75, -19.75) -> (19.75, 19.75) construction
  line L7 (19.75, 19.75) -> (-19.75, 19.75) construction
  line L8 (-19.75, 19.75) -> (19.75, -19.75) construction
  line L9 (-19.75, -19.75) -> (19.75, 19.75) construction
  point P0 (0, 0)
  dimension "d74" = 39.5
  dimension "d75" = 39.5
  constraints: 12 end point, 4 coincident, 2 midpoint, 2 parallel, 1 perpendicular, 1 vertical
  measures "d74" distance of L5.end L6.end
  measures "d75" distance of L6.end L4.start
hole "Hole1" at (-19.75, 19.75, -15) at (-19.75, -19.75, -15) at (19.75, -19.75, -15) at (19.75, 19.75, -15) direction (0, 0, 1) diameter 1.6942 end through all thread size "2-56 UNC" class "3B" standard "ANSI Unified Screw Threads"
sketch "Sketch14" plane through (-25, 25, -15) normal (0, 1, 0) x (1, 0, 0)
  line L0 (50, -32) -> (0, -32) projected
  line L1 (50, 0) -> (50, -32) projected
  line L2 (0, 0) -> (50, 0) projected
  line L3 (0, 0) -> (0, -32) projected
  line L4 (50, 0) -> (0, 0) construction
  line L5 (0, 0) -> (0, -32) construction
  line L6 (50, 0) -> (0, -32) construction
  line L7 (50, -32) -> (0, 0) construction
  line L8 (36.547, -16) -> (30.7735, -26)
  line L9 (30.7735, -26) -> (19.2265, -26)
  line L10 (19.2265, -26) -> (13.453, -16)
  line L11 (13.453, -16) -> (19.2265, -6)
  line L12 (19.2265, -6) -> (30.7735, -6)
  line L13 (30.7735, -6) -> (36.547, -16)
  point P0 (25, -15)
  point P1 (25, -16)
  dimension "d101" = 20
  constraints: 16 end point, 1 horizontal, 13 other
  measures "d101" distance between parallel lines of L9 L12
sketch "Sketch15" plane through (-25, 25, -15) normal (0, 1, 0) x (1, 0, 0)
  line L0 (0, 0) -> (50, 0) projected
  line L1 (50, 0) -> (50, -32) projected
  line L2 (50, -32) -> (0, -32) projected
  line L3 (0, 0) -> (0, -32) projected
  line L4 (0, 0) -> (50, -32) construction
  line L5 (50, 0) -> (0, -32) construction
  line L6 (13.1, -27.9) -> (36.9, -27.9) construction
  line L7 (36.9, -27.9) -> (36.9, -4.1) construction
  line L8 (36.9, -4.1) -> (13.1, -4.1) construction
  line L9 (13.1, -4.1) -> (13.1, -27.9) construction
  line L10 (13.1, -27.9) -> (36.9, -4.1) construction
  line L11 (36.9, -27.9) -> (13.1, -4.1) construction
  point P0 (25, -15)
  point P1 (25, -16)
  dimension "d93" = 23.8
  constraints: 16 end point, 4 coincident, 3 midpoint, 2 parallel, 2 perpendicular, 1 horizontal
  measures "d93" distance of L8.end L6.start
hole "Hole3" at (-11.9, 25, -10.9) at (11.9, 25, -10.9) at (11.9, 25, 12.9) at (-11.9, 25, 12.9) direction (0, -1, 0) diameter 1.6942 depth 4 thread size "2-56 UNC" class "2B" standard "ANSI Unified Screw Threads"
extrude "Extrusion13" cut sketch "Sketch14" against normal through all contours L8 L9 L10 L11 L12 L13
equation "\"d46\" = screwSpacing"
equation "\"d47\" = screwSpacing"
equation "\"d48\" = holeDiameter"
equation "\"d49\" = interiorWidth"
equation "\"d50\" = interiorWidth"
equation "\"d51\" = sideWallThickness"
equation "\"d52\" = sideWallThickness"
equation "\"d101\" = hexCoolingHole"
equation "\"screwSpacing\" = 34"
equation "\"interiorWidth\" = 42"
equation "\"bottomWallThickness\" = 2"
equation "\"holeDiameter\" = 1.8"
equation "\"sideWallThickness\" = 4"
equation "\"hexCoolingHole\" = 20"
body "Solid4"
body "Solid5"
